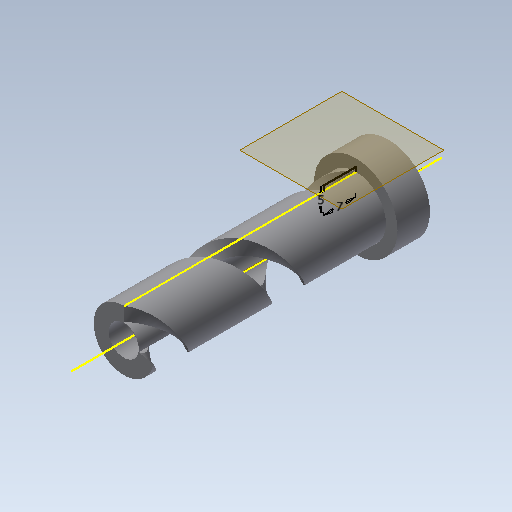
# Autodesk Inventor part: ScrewActuatorGripper
Saved by Autodesk Inventor 2020.1 (Build 241239000, 239)
## iProperties
Created: 2016-10-16
Part Number: ScrewActuatorGripper
Material: Generic
Document SubType Name: Modeling
Designer: Bardo91
Density: 1 g/cm^3
Appearance: Default
Author: Bardo91
Autodesk Inventor part; units mm, degrees
ref_plane "YZ Plane" through (0, 0, 0) normal (1, 0, 0) x (0, 1, 0)
ref_plane "XY Plane" through (0, 0, 0) normal (0, 0, 1) x (1, 0, 0)
sketch "Sketch1" plane through (0, 0, 0) normal (0, 0, 1) x (1, 0, 0)
  line L0 (0, 0) -> (0, 6)
  circle A0 centre (0, 6) radius 1.5
  circle A1 centre (-4.2426, 4.2426) radius 1.5
  circle A2 centre (-6, 0) radius 1.5
  circle A3 centre (-4.2426, -4.2426) radius 1.5
  circle A4 centre (0, -6) radius 1.5
  circle A5 centre (4.2426, -4.2426) radius 1.5
  circle A6 centre (6, 0) radius 1.5
  circle A7 centre (4.2426, 4.2426) radius 1.5
  circle A8 centre (0, 0) radius 9
  dimension "d0" = 6
  dimension "d1" = 3
  dimension "d4" = 360
  dimension "d6" = 18
  constraints: 9 centre point, 2 coincident, 2 end point, 1 vertical, 17 other
  measures "d0" distance of L0.start L0.end
  measures "d1" diameter of A0
  measures "d6" diameter of A8
extrude "Extrusion1" add sketch "Sketch1" along normal blind 7 contours A1 | A3 | A5 | A7 | A8
sketch "Sketch2" plane through (0, 0, 0) normal (0, 0, -1) x (-1, 0, 0)
  circle A0 centre (0, 0) radius 6.5
  dimension "d9" = 13
  constraints: 1 centre point, 1 coincident
  measures "d9" diameter of A0
extrude "Extrusion2" cut sketch "Sketch2" against normal blind 1
sketch "Sketch3" plane through (0, 0, 7) normal (0, 0, 1) x (1, 0, 0)
  circle A0 centre (0, 0) radius 6.5
  dimension "d12" = 13
  constraints: 1 centre point, 1 coincident
  measures "d12" diameter of A0
extrude "Extrusion3" add sketch "Sketch3" along normal blind 50
sketch "Sketch5" plane through (0, 0, 57) normal (0, 0, 1) x (1, 0, 0)
  circle A0 centre (0, 0) radius 3.25
  dimension "d25" = 6.5
  constraints: 1 centre point, 1 coincident
  measures "d25" diameter of A0
extrude "Extrusion5" cut sketch "Sketch5" against normal up to surface (56 mm away)
ref_plane "Work Plane1" through (0, 12, 0) normal (0, 1, 0) x (-1, 0, 0)
sketch "Sketch8" plane through (0, 0, 7) normal (0, 0, 1) x (1, 0, 0)
  circle A0 centre (0, 0) radius 3
  dimension "d44" = 6
  constraints: 1 centre point, 1 coincident
  measures "d44" diameter of A0
extrude "Extrusion8" cut sketch "Sketch8" against normal through all
sketch "Sketch9" plane through (0, 0, 0) normal (1, 0, 0) x (0, 1, 0)
  line L0 (6.5, 7) -> (6.5, 57) projected
  line L1 (6.5, 7) -> (6.5, 57) projected
  line L2 (6.3333, 7) -> (7.5, 7) projected
  line L3 (7.5, 7) -> (2.5, 7)
  line L4 (2.5, 7) -> (2.5, 14)
  line L5 (2.5, 14) -> (7.5, 14)
  line L6 (7.5, 14) -> (7.5, 7)
  line L7 (0, -11.4) -> (0, 68.4) projected
  point P0 (0, 0)
  dimension "d61" = 5
  dimension "d62" = 7
  constraints: 8 end point, 2 parallel, 1 horizontal, 1 perpendicular
  measures "d61" distance of L4.end L5.end
  measures "d62" distance of L3.end L4.end
coil "Coil2" sketch "Sketch9" operation cut axis through (0, 0, 7) along (0, 0, 1) pitch 25 turns 2 hand right taper 1
sketch "Boceto13" plane through (0, 0, 0) normal (0, 0, -1) x (-1, 0, 0)
  arc A0 (-6.3333, 1.4625) -> (-6.3333, -1.4625) centre (-6, 0) ccw projected
  circle A1 centre (-6, 0) radius 1.5
  arc A2 (-1.4625, -6.3333) -> (1.4625, -6.3333) centre (0, -6) ccw projected
  circle A3 centre (0, -6) radius 1.5
  arc A4 (1.4625, 6.3333) -> (-1.4625, 6.3333) centre (0, 6) ccw projected
  circle A5 centre (0, 6) radius 1.5
  arc A6 (6.3333, -1.4625) -> (6.3333, 1.4625) centre (6, 0) ccw projected
  circle A7 centre (6, 0) radius 1.5
  point P0 (0, 0)
  constraints: 4 centre point, 4 coincident
extrude "Extrusión9" add sketch "Boceto13" against normal blind 7
sketch "Boceto14" plane through (0, 0, 1) normal (0, 0, -1) x (-1, 0, 0)
  circle A0 centre (0, 0) radius 6.5
  constraints: 1 centre point, 1 coincident
extrude "Extrusión10" cut sketch "Boceto14" along normal blind 2
body "Solid1"
